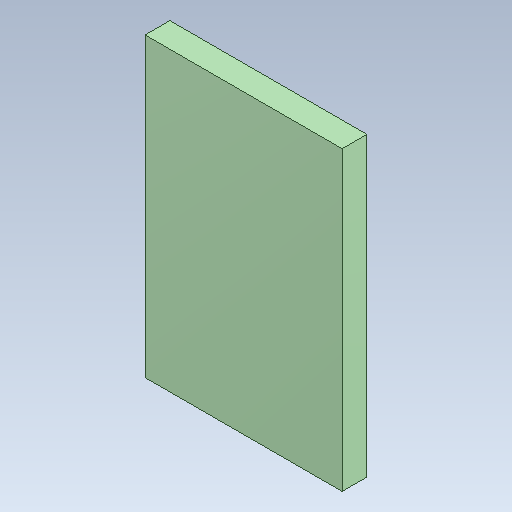
# Autodesk Inventor part: SPD30P06PTO252
Saved by Autodesk Inventor 2021 (Build 250183000, 183)
## iProperties
Created: 2020-11-18
Part Number: SPD30P06PTO252
Material: Generic
Document SubType Name: Modeling
Designer: Admin
Density: 1 g/cm^3
Appearance: TO252, SPD30P06PTO252
Author: Admin
Autodesk Inventor part; units mm, degrees
ref_plane "YZ Plane" through (0, 0, 0) normal (1, 0, 0) x (0, 1, 0)
ref_plane "XZ Plane" through (0, 0, 0) normal (0, 1, 0) x (-1, 0, 0)
ref_plane "XY Plane" through (0, 0, 0) normal (0, 0, 1) x (1, 0, 0)
sketch "TO252, SPD30P06PTO252_31" plane through (0, 0, 0) normal (0, 0, 1) x (1, 0, 0)
  line L0 (-3.973, 5.983) -> (3.973, 5.983)
  line L1 (3.973, 5.983) -> (3.973, -5.983)
  line L2 (3.973, -5.983) -> (-3.973, -5.983)
  line L3 (-3.973, -5.983) -> (-3.973, 5.983)
  constraints: 8 end point
extrude "Extrusion1" add sketch "TO252, SPD30P06PTO252_31" along normal blind 1
body "Solid1"
